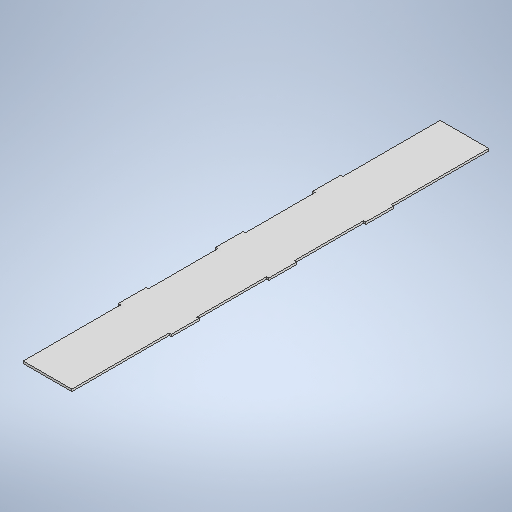
# Autodesk Inventor part: Trebuchet V1 - Runway
Saved by Autodesk Inventor 2025.2 (Build 292293000, 293)
## iProperties
Created: 2025-04-07
Part Number: Trebuchet V1 - Runway
Material: Generic
Document SubType Name: Modeling
Designer: Dylan
Density: 1 g/cm^3
Appearance: Default
Author: VRK99-0110
Title: Trebuchet - Runway
Subject: Trebuchet Project
Autodesk Inventor part; units mm, degrees
ref_plane "YZ Plane" through (0, 0, 0) normal (1, 0, 0) x (0, 1, 0)
ref_plane "XZ Plane" through (0, 0, 0) normal (0, 1, 0) x (-1, 0, 0)
ref_plane "XY Plane" through (0, 0, 0) normal (0, 0, 1) x (1, 0, 0)
sketch "Sketch1" plane through (0, 0, 0) normal (0, 1, 0) x (-1, 0, 0)
  line L0 (0, 0) -> (0, -600)
  line L1 (0, -600) -> (70, -600)
  line L2 (70, -600) -> (70, 0)
  line L3 (70, 0) -> (0, 0)
  line L4 (0, 0) -> (0, -300)
  line L5 (-3.2, -280) -> (-3.2, -320)
  line L6 (-3.2, -320) -> (0, -320)
  line L7 (-3.2, -280) -> (0, -280)
  line L8 (-3.2, -420) -> (0, -420)
  line L9 (-3.2, -420) -> (-3.2, -460)
  line L10 (-3.2, -460) -> (0, -460)
  line L11 (-3.2, -180) -> (0, -180)
  line L12 (-3.2, -180) -> (-3.2, -140)
  line L13 (-3.2, -140) -> (0, -140)
  line L14 (73.2, -280) -> (73.2, -320)
  line L15 (73.2, -320) -> (70, -320)
  line L16 (73.2, -280) -> (70, -280)
  line L17 (73.2, -420) -> (70, -420)
  line L18 (73.2, -420) -> (73.2, -460)
  line L19 (73.2, -460) -> (70, -460)
  line L20 (73.2, -180) -> (70, -180)
  line L21 (73.2, -180) -> (73.2, -140)
  line L22 (73.2, -140) -> (70, -140)
  dimension "d0" = 600
  dimension "d2" = 70
  dimension "d3" = 600
  dimension "d7" = 40
  dimension "d8" = 100
  dimension "d9" = 40
  dimension "d10" = 100
  dimension "d11" = 40
  constraints: 46 end point, 7 perpendicular, 6 point on line, 3 vertical, 1 horizontal, 1 midpoint
  measures "d0" distance of L0.start L0.end
  measures "d2" distance of L0.end L1.end
  measures "d3" distance of L1.end L2.end
  measures "d7" distance of L5.start L5.end
  measures "d8" distance of L5.end L8.start
  measures "d9" distance of L8.start L9.end
  measures "d10" distance of L5.start L11.start
  measures "d11" distance of L11.start L12.end
extrude "Extrusion1" add sketch "Sketch1" along normal blind 3.175
body "Solid1"
